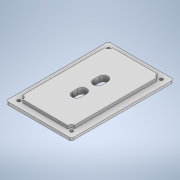
# Autodesk Inventor part: tampa
Saved by Autodesk Inventor 2022 (Build 260153000, 153)
## iProperties
Created: 2022-03-11
Part Number: tampa
Material: Genérico
Document SubType Name: Modeling
Designer: Guilherme
Density: 1 g/cm^3
Appearance: Padrão
Author: Guilherme
Autodesk Inventor part; units mm, degrees
ref_plane "YZ Plane" through (0, 0, 0) normal (1, 0, 0) x (0, 1, 0)
ref_plane "XZ Plane" through (0, 0, 0) normal (0, 1, 0) x (-1, 0, 0)
ref_plane "XY Plane" through (0, 0, 0) normal (0, 0, 1) x (1, 0, 0)
sketch "Esboço1" plane through (0, 0, 0) normal (0, 1, 0) x (-1, 0, 0)
  line L0 (-34, 53) -> (34, 53)
  line L1 (34, 53) -> (34, -53)
  line L2 (34, -53) -> (-34, -53)
  line L3 (-34, -53) -> (-34, 53)
  line L4 (-34, 53) -> (34, -53) construction
  line L5 (34, 53) -> (-34, -53) construction
  point P0 (0, 0)
  dimension "d0" = 68
  dimension "d1" = 106
  constraints: 12 end point, 2 midpoint, 2 parallel, 1 horizontal, 1 perpendicular
  measures "d0" distance of L1.end L2.end
  measures "d1" distance of L0.end L1.end
extrude "Extrusão1" add sketch "Esboço1" along normal blind 3
sketch "Esboço4" plane through (0, 3, 0) normal (0, 1, 0) x (1, 0, 0)
  line L0 (29.972, -49.0345) -> (-29.972, -49.0345)
  line L1 (-29.972, -49.0345) -> (-29.972, 49.0345)
  line L2 (-29.972, 49.0345) -> (29.972, 49.0345)
  line L3 (29.972, 49.0345) -> (29.972, -49.0345)
  line L4 (29.972, -49.0345) -> (-29.972, 49.0345) construction
  line L5 (-29.972, -49.0345) -> (29.972, 49.0345) construction
  circle A0 centre (-27.305, -46.4815) radius 1.6765
  circle A1 centre (27.305, -46.4815) radius 1.6765
  circle A2 centre (-27.305, 46.4825) radius 1.6765
  circle A3 centre (27.305, 46.4825) radius 1.6765
  point P0 (0, 0)
  dimension "d11" = 59.944
  dimension "d12" = 98.069
  dimension "d13" = 3.353
  dimension "d14" = 2.667
  dimension "d15" = 2.553
  dimension "d18" = 54.61
  dimension "d21" = 92.964
  constraints: 12 end point, 4 centre point, 2 horizontal, 2 midpoint, 2 parallel, 1 perpendicular, 1 vertical, 6 other
  measures "d11" distance of L1.end L2.end
  measures "d12" distance of L0.end L1.end
  measures "d13" diameter of A0
  measures "d14" distance from line of L1 A0.centre
  measures "d15" distance from line of L0 A0.centre
  measures "d18" distance of A0.centre A1.centre
  measures "d21" distance of A0.centre A2.centre
extrude "Extrusão3" cut sketch "Esboço4" against normal blind 3 contours A0 | A1 | A2 | A3
sketch "Esboço5" plane through (0, 3, 0) normal (0, 1, 0) x (1, 0, 0)
  circle A0 centre (-27.305, -46.4815) radius 1.6765 projected
  arc A1 (-23.305, -46.4825) -> (-27.305, -42.4815) centre (-27.305, -46.4815) ccw
  circle A2 centre (27.305, -46.4815) radius 1.6765 projected
  arc A3 (26.645, -42.5363) -> (23.305, -46.4825) centre (27.305, -46.4815) ccw
  circle A4 centre (27.305, 46.4825) radius 1.6765 projected
  arc A5 (23.305, 46.4825) -> (26.645, 42.5373) centre (27.305, 46.4825) ccw
  circle A6 centre (-27.305, 46.4825) radius 1.6765 projected
  arc A7 (-27.305, 42.4825) -> (-23.305, 46.4825) centre (-27.305, 46.4825) ccw
  line L0 (26.645, 42.5373) -> (26.645, -42.5363)
  line L1 (27.1364, -46.1956) -> (-27.305, 46.4825) construction
  line L2 (-26.975, -46.4825) -> (26.975, 46.4825) construction
  line L3 (-27.305, -42.4815) -> (-27.305, 42.4825)
  line L4 (23.305, -46.4825) -> (-23.305, -46.4825)
  line L5 (-23.305, 46.4825) -> (23.305, 46.4825)
  point P0 (0, 0)
  dimension "d26" = 8
  dimension "d27" = 8
  dimension "d28" = 8
  dimension "d29" = 8
  constraints: 12 end point, 8 point on circle, 4 centre point, 4 coincident, 2 parallel, 1 horizontal, 1 midpoint, 1 perpendicular, 1 point on line
  measures "d26" diameter of A1
  measures "d27" diameter of A3
  measures "d28" diameter of A5
  measures "d29" diameter of A7
extrude "Extrusão4" add sketch "Esboço5" along normal blind 3 contours A1 L3 A7 L5 A5 L0 A3 L4
sketch "Esboço7" plane through (-34, 0, 53) normal (0, 0, 1) x (1, 0, 0)
  line L0 (68, 0) -> (68, 3) projected
  line L1 (68, 0) -> (68, 3)
  line L2 (68, 3) -> (67.4537, -0.098)
  line L3 (67.4537, -0.098) -> (68, -0.098)
  line L4 (68, 0) -> (0, 0) projected
  line L5 (68, -0.098) -> (68, 0)
  line L6 (68, 3) -> (0, 3) projected
  line L7 (68, 0) -> (68, 3)
  point P0 (34, 0)
  dimension "d36" = 10
  constraints: 10 end point, 3 perpendicular, 1 collinear, 1 point on line
  measures "d36" angle of L2 L1
extrude "Extrusão6" cut sketch "Esboço7" against normal blind 114
fillet "Arredondamento1" radius 2 4 edges at (-34, 1.5, 53) (33.7355, 1.5, 53) (-34, 1.5, -53) (33.7355, 1.5, -53)
sketch "Esboço8" plane through (0, 6, 0) normal (0, 1, 0) x (1, 0, 0)
  arc A0 (4.65, 14) -> (-4.65, 14) centre (0, 14) ccw
  arc A1 (-4.65, 8) -> (4.65, 8) centre (0, 8) ccw
  arc A2 (4.65, -8) -> (-4.65, -8) centre (0, -8) ccw
  arc A3 (-4.65, -14) -> (4.65, -14) centre (0, -14) ccw
  line L0 (4.65, 14) -> (4.65, 8)
  line L1 (-4.65, 14) -> (-4.65, 8)
  line L2 (4.65, -8) -> (4.65, -14)
  line L3 (-4.65, -14) -> (-4.65, -8)
  point P0 (0, 0)
  dimension "d40" = 9.3
  dimension "d41" = 9.3
  dimension "d42" = 9.3
  dimension "d43" = 9.3
  dimension "d44" = 6
  dimension "d45" = 6
  dimension "d46" = 8
  dimension "d47" = 8
  constraints: 8 end point, 8 point on circle, 4 centre point, 4 point on line, 2 tangent
  measures "d40" diameter of A0
  measures "d41" diameter of A1
  measures "d42" diameter of A2
  measures "d43" diameter of A3
  measures "d44" distance of A1.centre A0.centre
  measures "d45" distance of A3.centre A2.centre
  measures "d46" distance of point (0, 0) A1.centre
  measures "d47" distance of point (0, 0) A2.centre
extrude "Extrusão7" cut sketch "Esboço8" against normal blind 10
